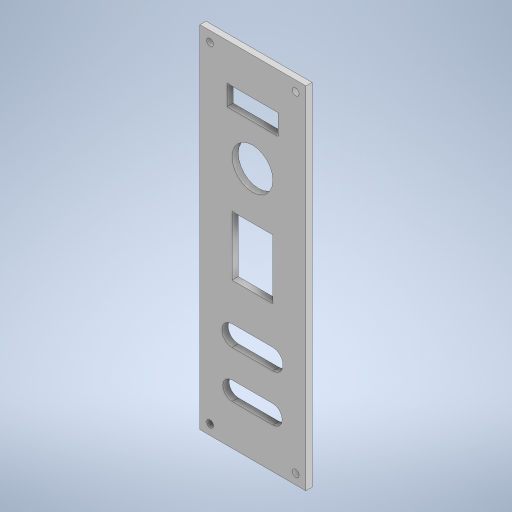
# Autodesk Inventor part: port plugin
Saved by Autodesk Inventor 2023 (Build 270158030, 158C)
## iProperties
Created: 2023-03-06
Part Number: port plugin
Material: Generic
Document SubType Name: Modeling
Designer: fatih
Density: 1 g/cm^3
Appearance: Default
Author: fatih
Autodesk Inventor part; units mm, degrees
ref_plane "YZ Plane" through (0, 0, 0) normal (1, 0, 0) x (0, 1, 0)
ref_plane "XZ Plane" through (0, 0, 0) normal (0, 1, 0) x (-1, 0, 0)
ref_plane "XY Plane" through (0, 0, 0) normal (0, 0, 1) x (1, 0, 0)
sketch "Sketch1" plane through (0, 0, 0) normal (0, 0, 1) x (1, 0, 0)
  line L0 (0, 0) -> (52, 0)
  line L1 (52, 0) -> (52, 172)
  line L2 (52, 172) -> (0, 172)
  line L3 (0, 172) -> (0, 0)
  line L4 (0, 0) -> (10, 0)
  line L5 (10, 0) -> (10, 10)
  line L6 (10, 10) -> (0, 10)
  line L7 (0, 10) -> (0, 0)
  circle A0 centre (5, 5) radius 1.7
  line L8 (52, 0) -> (42, 0)
  line L9 (42, 0) -> (42, 10)
  line L10 (42, 10) -> (52, 10)
  line L11 (52, 10) -> (52, 0)
  circle A1 centre (47, 5) radius 1.7
  line L12 (52, 86) -> (47, 86)
  line L13 (0, 172) -> (10, 172)
  line L14 (10, 172) -> (10, 162)
  line L15 (10, 162) -> (0, 162)
  line L16 (0, 162) -> (0, 172)
  circle A2 centre (5, 167) radius 1.7
  line L17 (52, 172) -> (42, 172)
  line L18 (42, 172) -> (42, 162)
  line L19 (42, 162) -> (52, 162)
  line L20 (52, 162) -> (52, 172)
  circle A3 centre (47, 167) radius 1.7
  dimension "d0" = 52
  dimension "d1" = 172
  dimension "d2" = 10
  dimension "d3" = 10
  dimension "d4" = 3.4
  constraints: 42 end point, 8 symmetric about line, 4 centre point, 4 parallel, 3 horizontal, 2 perpendicular, 1 midpoint, 2 other
  measures "d0" distance of L1.end L2.end
  measures "d1" distance of L2.end L0.start
  measures "d2" distance of L6.end L5.end
  measures "d3" distance of L5.end L4.end
  measures "d4" diameter of A0
extrude "Extrusion1" add sketch "Sketch1" along normal blind 3
sketch "Sketch2" plane through (0, 0, 3) normal (0, 0, 1) x (1, 0, 0)
  circle A0 centre (5, 167) radius 1.7 projected
  circle A1 centre (47, 5) radius 1.7 projected
  line L0 (5, 167) -> (47, 167)
  line L1 (47, 167) -> (47, 5)
  line L2 (47, 5) -> (5, 5)
  line L3 (5, 5) -> (5, 167)
  line L4 (13.3003, 153.806) -> (38.3003, 153.806)
  line L5 (38.3003, 153.806) -> (38.3003, 143.806)
  line L6 (38.3003, 143.806) -> (13.3003, 143.806)
  line L7 (13.3003, 143.806) -> (13.3003, 153.806)
  circle A2 centre (25.8003, 123.7951) radius 10
  line L8 (35.8003, 86) -> (35.8003, 100.6048)
  line L9 (35.8003, 100.6048) -> (26, 100.6048)
  line L10 (35.8003, 100.6048) -> (15.8003, 100.6048)
  line L11 (15.8003, 100.6048) -> (15.8003, 71.4048)
  line L12 (15.8003, 71.4048) -> (35.8003, 71.4048)
  line L13 (35.8003, 71.4048) -> (35.8003, 100.6048)
  line L14 (15.8003, 47.8583) -> (35.8003, 47.8583) construction
  line L15 (15.8003, 52.8601) -> (35.8003, 52.8601)
  line L16 (35.8003, 42.8565) -> (15.8003, 42.8565)
  arc A3 (15.8003, 52.8601) -> (15.8003, 42.8565) centre (15.8003, 47.8583) ccw
  arc A4 (35.8003, 42.8565) -> (35.8003, 52.8601) centre (35.8003, 47.8583) ccw
  line L17 (15.8003, 24.4407) -> (35.8003, 24.4407) construction
  line L18 (15.8003, 19.8936) -> (35.8003, 19.8936)
  line L19 (35.8003, 28.9878) -> (15.8003, 28.9878)
  arc A5 (15.8003, 28.9878) -> (15.8003, 19.8936) centre (15.8003, 24.4407) ccw
  arc A6 (35.8003, 19.8936) -> (35.8003, 28.9878) centre (35.8003, 24.4407) ccw
  point P0 (0, 0)
  point P1 (25.8003, 47.8583)
  point P2 (25.8003, 24.4407)
  dimension "d7" = 25
  dimension "d8" = 10
  dimension "d9" = 20
  dimension "d10" = 29.2
  constraints: 44 end point, 9 parallel, 8 point on circle, 8 tangent, 5 centre point, 4 horizontal, 3 perpendicular, 2 midpoint
  measures "d7" distance of L5.end L6.end
  measures "d8" distance of L4.end L5.end
  measures "d9" diameter of A2
  measures "d10" distance of L11.end L10.end
extrude "Extrusion2" cut sketch "Sketch2" against normal blind 3 contours L4 L5 L6 L7 | A2 | L13 L12 L11 L10 L9 L8 | L15 A4 L16 A3 | A5 L19 A6 L18
body "Solid1"
